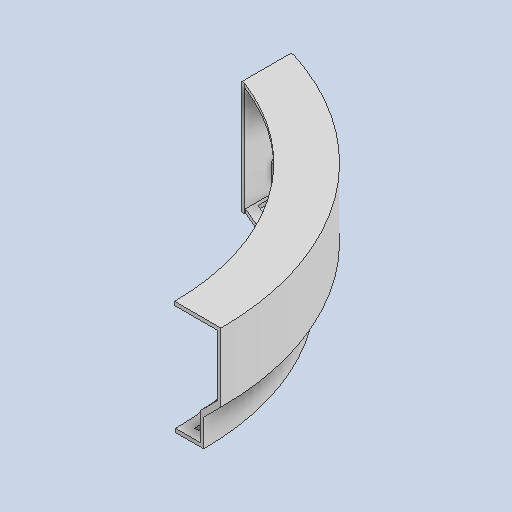
# Autodesk Inventor part: Bottom_Enclosure_1_v2_MIRROR
Saved by Autodesk Inventor 2026 (Build 300175050, 175E)
## iProperties
Created: 2026-01-05
Part Number: Bottom_Enclosure_1_v2_MIRROR
Material: Generic
Document SubType Name: Modeling
Designer: Kartik
Mass: 134.386 g
Surface Area: 913 cm^2
Volume: 134.386 cm^3
Density: 1 g/cm^3
Appearance: Default
Author: Kartik
Autodesk Inventor part; units mm, degrees
ref_plane "YZ Plane" through (0, 0, 0) normal (1, 0, 0) x (0, 1, 0)
ref_plane "XZ Plane" through (0, 0, 0) normal (0, 1, 0) x (-1, 0, 0)
ref_plane "XY Plane" through (0, 0, 0) normal (0, 0, 1) x (1, 0, 0)
sketch "Sketch1" plane through (0, 0, 0) normal (0, 0, 1) x (1, 0, 0)
  line L0 (0, 0) -> (3, 0)
  line L1 (3, 0) -> (3, 22.5)
  line L2 (3, 22.5) -> (17.1421, 36.6421)
  line L3 (17.1421, 36.6421) -> (17.1421, 92.6421)
  line L4 (17.1421, 92.6421) -> (14.1421, 92.6421)
  line L5 (17.1421, 36.6421) -> (10.8717, 42.9126)
  line L6 (14.1421, 92.6421) -> (14.1421, 39.6421)
  line L7 (3, 22.5) -> (-2.0059, 27.5059)
  line L8 (14.1421, 39.6421) -> (0, 25.5)
  line L9 (0, 25.5) -> (0, 0)
  line L10 (0, 0) -> (-20, 0)
  line L11 (-20, 0) -> (-20, 3)
  line L12 (-20, 3) -> (0, 3)
  line L13 (0, 3) -> (0, 0)
  line L14 (14.1421, 92.6421) -> (-20.8579, 92.6421)
  line L15 (-20.8579, 92.6421) -> (-20.8579, 89.6421)
  line L16 (-20.8579, 89.6421) -> (14.1421, 89.6421)
  line L17 (14.1421, 89.6421) -> (14.1421, 92.6421)
  point P0 (14.1421, 89.6421)
  dimension "d0" = 3
  dimension "d1" = 22.5
  dimension "d2" = 20
  dimension "d3" = 135
  dimension "d4" = 56
  dimension "d5" = 3
  dimension "d9" = 20
  dimension "d10" = 3
  dimension "d11" = 35
  dimension "d12" = 3
  constraints: 36 end point, 5 parallel, 5 perpendicular, 3 horizontal, 2 point on line, 2 vertical
  measures "d0" distance of L0.start L0.end
  measures "d1" distance of L0.end L1.end
  measures "d2" distance of L1.end L2.end
  measures "d3" angle of L1 L2
  measures "d4" distance of L2.end L3.end
  measures "d5" distance of L3.end L4.end
  measures "d9" distance of L11.end L12.end
  measures "d10" distance of L10.end L11.end
  measures "d11" distance of L16.end L15.end
  measures "d12" distance of L15.end L14.end
sketch "Sketch2" plane through (0, 0, 0) normal (0, 1, 0) x (-1, 0, 0)
  circle A0 centre (217, 0) radius 220
  point P0 (0, 0)
  point P1 (-3, 0)
  point P2 (-3, 0)
  point P3 (-3, 0)
  dimension "d6" = 440
  constraints: 1 horizontal alignment, 2 other
sketch "Sketch3" plane through (0, 0, 0) normal (0, 0, 1) x (1, 0, 0)
  line L0 (-217, 0) -> (-217, 100)
  point P0 (0, 0)
  dimension "d7" = 100
  constraints: 2 end point, 1 vertical
  measures "d7" distance of L0.start L0.end
revolve "Revolution1" add sketch "Sketch1" angle 90 about axis through (-217, 0, 0) along (0, 1, 0)
sketch "Sketch4" plane through (-20.8579, 92.6421, 0) normal (0, 1, 0) x (1, 0, 0)
  line L0 (-196.1421, 196.1421) -> (-196.1421, 234.1421) projected
  line L1 (-126.1421, 196.1421) -> (-126.1421, 234.1421)
  line L2 (-196.1421, 234.1421) -> (-153.5416, 245.1684)
  line L3 (-153.5416, 245.1684) -> (-126.1421, 234.1421)
  line L4 (-126.1421, 196.1421) -> (-126.1421, 171.9563)
  line L5 (-126.1421, 171.9563) -> (-196.1421, 196.1421)
  point P0 (20.8579, 0)
  dimension "d13" = 70
  constraints: 10 end point, 1 parallel, 1 vertical
  measures "d13" distance between parallel lines of L0 L1
extrude "Extrusion1" cut sketch "Sketch4" against normal through all
sketch "Sketch5" plane through (-147, 92.6421, -223.4335) normal (-1, 0, 0) x (0, 0, 1)
  line L0 (0, 0) -> (40.2076, 0) projected
  line L1 (0, -56) -> (0, 0) projected
  spline S0 degree 2 poles (14.867, -70.1421) (7.665, -63.3144) (0, -56) knots 0 0 0 1 1 1 weights 1 1.000536 1 projected
  line L2 (14.867, -92.6421) -> (14.867, -70.1421) projected
  line L3 (39.2896, -92.6421) -> (14.867, -92.6421) projected
  line L4 (40.2076, 0) -> (40.2076, -92.6421)
  line L5 (223.4335, -56) -> (0, -56) projected
  line L6 (40.2076, -92.6421) -> (38.6722, -92.6421)
  point P0 (223.4335, -92.6421)
  constraints: 4 end point, 1 perpendicular, 1 point on line, 1 other
extrude "Extrusion2" add sketch "Sketch5" along normal blind 2
ref_plane "Work Plane1" through (14.1421, 39.6421, 0) normal (0.7071068, -0.7071068, 0) x (0.7071068, 0.7071068, 0)
sketch "Sketch6" plane through (14.1421, 39.6421, 0) normal (0.7071068, -0.7071068, 0) x (0.7071068, 0.7071068, 0)
  line L0 (0, 0) -> (-20, 0) projected
  ellipse E0 centre (-173.4422, 0) end of major axis (-173.4422, -217) minor radius 153.4422 (-123.9447, -205.3996) -> (-20, 0) ccw projected
  ellipse E1 centre (-163.4422, 0) end of major axis (-163.4422, -231.1421) minor radius 163.4422 (-113.9447, -220.2877) -> (0, 0) ccw projected
  circle A0 centre (-34.9129, -120.4469) radius 8
  circle A1 centre (-46.3311, -142.6871) radius 8
  line L1 (-34.9129, -120.4469) -> (-46.3311, -142.6871)
  circle A2 centre (-40.622, -131.567) radius 12.5
  point P0 (-38.0312, 0)
  dimension "d22" = 25
  dimension "d18" = 16
  dimension "d19" = 16
  constraints: 2 centre point, 2 end point, 1 midpoint, 5 other
  measures "d18" diameter of A0
  measures "d19" diameter of A1
extrude "Extrusion3" [suppressed]
sketch "Sketch7" plane through (-20, 0, 0) normal (0, -1, 0) x (1, 0, 0)
  arc A0 (-127, -208.5665) -> (23, 0) centre (-197, 0) ccw projected
  arc A1 (-127, -184.144) -> (0, 0) centre (-197, 0) ccw projected
  line L0 (0, 0) -> (23, 0) projected
  arc A2 (-124.1574, -199.0928) -> (14.849, -8) centre (-197, 0) ccw
  line L1 (14.849, -8) -> (7.8438, -8)
  arc A3 (-124.1574, -191.6219) -> (7.8438, -8) centre (-197, 0) ccw
  line L2 (-124.1574, -191.6219) -> (-124.1574, -199.0928)
  point P0 (20, 0)
  dimension "d25" = 8
  constraints: 4 end point, 4 point on circle, 2 centre point, 1 vertical, 1 other
  measures "d25" distance between parallel lines of L0 L1
extrude "Extrusion4" cut sketch "Sketch7" against normal blind 10
ref_plane "Work Plane2" through (14.1421, 39.6421, 0) normal (0.6123724, -0.6123724, -0.5) x (-0.7071068, -0.7071068, 0)
sketch "Sketch8" plane through (14.1421, 39.6421, 0) normal (0.6123724, -0.6123724, -0.5) x (-0.7071068, -0.7071068, 0)
  ellipse E0 centre (173.4422, 76.7211) end of major axis (270.4875, 270.8118) minor radius 132.8848 (123.9447, 229.8536) -> (20, 0) ccw projected
  line L0 (0, 0) -> (20, 0) projected
  ellipse E1 centre (163.4422, 81.7211) end of major axis (266.8121, 288.4609) minor radius 141.5451 (113.9447, 247.7471) -> (0, 0) ccw projected
  circle A0 centre (26.5351, 91.9942) radius 8
  circle A1 centre (34.3492, 115.7416) radius 8
  line L1 (34.3492, 115.7416) -> (26.5351, 91.9942)
  circle A2 centre (30.4422, 103.8679) radius 12.5
  point P0 (38.0312, -9.0156)
  dimension "d31" = 25
  dimension "d29" = 16
  dimension "d30" = 16
  dimension "d32" = 133
  constraints: 2 centre point, 2 end point, 1 midpoint, 6 other
  measures "d29" diameter of A0
  measures "d30" diameter of A1
  measures "d32" horizontal distance of point (163.442, 81.721) point (30.442, 103.868)
extrude "Extrusion5" cut sketch "Sketch8" along normal up to surface contours A2 A1 | A1 L1 A2 | A2 L1 A0 | A0 A2 | A1 A2 L1 | L1 A2 A0 round surface about axis through (-217, 29.5711, 0) along (0, 1, 0) radius 227.0711 half angle 45 far side no
body "Solid1"
